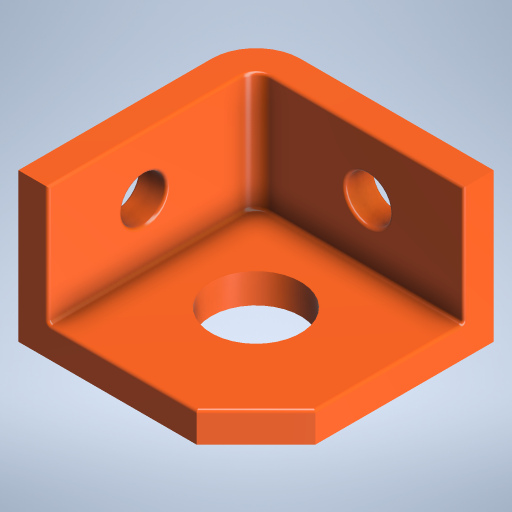
# Autodesk Inventor part: Tutorial Pt.1
Saved by Autodesk Inventor 2024.4 (Build 284460000, 460)
## iProperties
Created: 2026-06-11
Part Number: Tutorial Pt.1
Material: Stainless Steel
Document SubType Name: Modeling
Designer: stanc
Density: 8 g/cm^3
Appearance: Smooth - Light Orange
Author: stanc
Autodesk Inventor part; units mm, degrees
ref_plane "YZ Plane" through (0, 0, 0) normal (1, 0, 0) x (0, 1, 0)
ref_plane "XZ Plane" through (0, 0, 0) normal (0, 1, 0) x (-1, 0, 0)
ref_plane "XY Plane" through (0, 0, 0) normal (0, 0, 1) x (1, 0, 0)
sketch "Sketch1" plane through (0, 0, 0) normal (0, 1, 0) x (-1, 0, 0)
  line L0 (0, 0) -> (80, 0)
  line L1 (80, 0) -> (80, -80)
  line L2 (80, -80) -> (0, -80)
  line L3 (0, -80) -> (0, 0)
  circle A0 centre (40, -40) radius 15
  line L4 (20, 0) -> (0, -20)
  point P0 (80, -40)
  point P1 (40, -80)
  dimension "d0" = 80
  dimension "d1" = 80
  dimension "d3" = 30
  dimension "d4" = 20
  dimension "d5" = 20
  constraints: 10 end point, 2 midpoint, 2 parallel, 2 point on line, 1 centre point, 1 horizontal, 1 horizontal alignment, 1 perpendicular, 1 vertical alignment
  measures "d0" distance of L0.end L1.end
  measures "d1" distance of L0.start L0.end
  measures "d3" diameter of A0
  measures "d4" distance of L0.start L4.start
  measures "d5" distance of L0.start L4.end
extrude "Extrusion1" add sketch "Sketch1" along normal blind 10 contours L0 L1 L2 L3 L4
sketch "Sketch2" plane through (0, 10, 0) normal (0, 1, 0) x (1, 0, 0)
  line L0 (0, 80) -> (-80, 80) projected
  line L1 (0, 20) -> (0, 80) projected
  line L2 (-80, 80) -> (0, 80)
  line L3 (0, 80) -> (0, 70)
  line L4 (0, 70) -> (-80, 70)
  line L5 (-80, 70) -> (-80, 80)
  line L6 (-80, 80) -> (-80, 0) projected
  line L7 (-80, 0) -> (-70, 0)
  line L8 (-70, 0) -> (-70, 80)
  line L9 (-70, 80) -> (-80, 80)
  line L10 (-80, 80) -> (-80, 0)
  point P0 (0, 0)
  point P1 (-70, 70)
  dimension "d8" = 10
  dimension "d9" = 10
  constraints: 16 end point, 4 parallel, 2 horizontal, 2 perpendicular, 2 point on line
  measures "d8" distance between parallel lines of L4 L0
  measures "d9" distance between parallel lines of L6 L8
extrude "Extrusion2" add sketch "Sketch2" along normal blind 40
fillet "Fillet1" radius 5 1 edges at (-70, 30, -70)
fillet "Fillet2" radius 15 1 edges at (-80, 25, -80)
sketch "Sketch3" plane through (0, 10, -70) normal (0, 0, 1) x (1, 0, 0)
  circle A0 centre (-32.5, 20) radius 7.5
  line L0 (0, 0) -> (0, 40) projected
  line L1 (-65, 40) -> (0, 40) projected
  line L2 (-80, -10) -> (-80, 40) projected
  point P0 (0, -10)
  point P1 (0, 20)
  point P2 (-32.5, 40)
  point P3 (-32.5, 40)
  point P4 (0, 20)
  point P5 (0, 20)
  point P6 (0, 20)
  dimension "d14" = 15
  dimension "d15" = 80
  constraints: 6 midpoint, 4 horizontal alignment, 2 vertical alignment, 1 centre point
  measures "d14" diameter of A0
  measures "d15" distance between parallel lines of L2 L0
extrude "Extrusion3" cut sketch "Sketch3" against normal blind 40
sketch "Sketch4" plane through (-70, 10, 0) normal (1, 0, 0) x (0, 0, -1)
  circle A0 centre (32.4993, 20) radius 7.5
  line L0 (65, 40) -> (65, 0) projected
  line L1 (0, 0) -> (0, 40) projected
  point P0 (0, -10)
  point P1 (0, 20)
  dimension "d18" = 15
  dimension "d19" = 65
  dimension "d20" = 32.4993
  constraints: 1 centre point, 1 horizontal alignment, 1 midpoint
  measures "d18" diameter of A0
  measures "d19" distance between parallel lines of L0 L1
  measures "d20" distance from line of A0.centre L1
extrude "Extrusion4" cut sketch "Sketch4" against normal blind 40
fillet "Fillet3" radius 1 14 edges at (-32.5, 50, -70) (-70, 50, -32.5) (-70, 30, 0) (-68.5355, 10, -68.5355) (-32.5, 10, -70) (-70, 10, -32.5) (-45, 10, 0) (-10, 10, -10) (0, 10, -45) (0, 30, -70) (-70, 30, -24.9993) (-40, 30, -70) (-40, 30, -80) (-80, 30, -24.9993)
body "Solid1"
